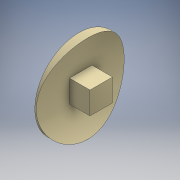
# Autodesk Inventor part: ET19
Saved by Autodesk Inventor 2016 (Build 200138000, 138)
## iProperties
Created: 2016-03-28
Part Number: ET19
Material: Genérico
Document SubType Name: Modeling
Designer: Usuario1
Density: 1 g/cm^3
Appearance: Valor por defecto
Author: Usuario1
Autodesk Inventor part; units mm, degrees
ref_plane "YZ Plane" through (0, 0, 0) normal (1, 0, 0) x (0, 1, 0)
ref_plane "XZ Plane" through (0, 0, 0) normal (0, 1, 0) x (-1, 0, 0)
ref_plane "XY Plane" through (0, 0, 0) normal (0, 0, 1) x (1, 0, 0)
sketch "Boceto1" plane through (0, 0, 0) normal (1, 0, 0) x (0, 1, 0)
  circle A0 centre (-0.0022, 0) radius 0.8492
  circle A1 centre (-1.5281, -0.0006) radius 0.1032
  circle A2 centre (0, 0) radius 0.9775
  constraints: 3 centre point
extrude "Extrusión1" add sketch "Boceto1" along normal blind 0.2 contours A0 | A2
sketch "Boceto2" plane through (0, 0, 0) normal (0, 1, 0) x (-1, 0, 0)
  arc A0 (-0.1981, -0.9764) -> (-0.1981, 0.9764) centre (-2.9972, 0) ccw
  arc A1 (-0.1981, 0.9764) -> (-0.4354, 1.174) centre (-0.4814, 0.8776) ccw
  arc A2 (-0.4354, -1.174) -> (-0.1981, -0.9764) centre (-0.4814, -0.8776) ccw
  arc A3 (-0.1981, -0.9764) -> (-0.1981, 0.9764) centre (-2.9972, 0) ccw
  arc A4 (-0.1981, 0.9764) -> (-0.4354, 1.174) centre (-0.4814, 0.8776) ccw
  arc A5 (-0.4354, -1.174) -> (-0.1981, -0.9764) centre (-0.4814, -0.8776) ccw
  arc A6 (-0.1981, -0.9764) -> (-0.1981, 0.9764) centre (-2.9972, 0) ccw
  arc A7 (-0.1981, 0.9764) -> (-0.4354, 1.174) centre (-0.4814, 0.8776) ccw
  arc A8 (-0.4354, -1.174) -> (-0.1981, -0.9764) centre (-0.4814, -0.8776) ccw
  line L0 (-0.2, 0.9775) -> (-0.2, -0.9775) projected
  line L1 (0, -0.9775) -> (0, 0.9775) projected
  line L2 (-0.4354, 1.174) -> (-0.4354, -1.174)
  point P0 (0, 0)
  constraints: 18 point on circle, 9 centre point, 2 end point, 1 vertical
extrude "Extrusión2" cut sketch "Boceto2" along normal mid plane 10
sketch "Boceto3" plane through (0, 0, 0) normal (-1, 0, 0) x (0, 0, 1)
  line L0 (0, 0) -> (0, -0.25)
  line L1 (0, -0.25) -> (-0.25, -0.25)
  line L2 (-0.25, -0.25) -> (-0.25, 0.25)
  line L3 (-0.25, 0.25) -> (0.25, 0.25)
  line L4 (0.25, 0.25) -> (0.25, -0.25)
  line L5 (0.25, -0.25) -> (-0.25, -0.25)
  dimension "d4" = 0.25
  dimension "d5" = 0.25
  dimension "d6" = 0.5
  dimension "d7" = 0.5
  dimension "d8" = 0.5
  constraints: 12 end point, 3 perpendicular, 1 point on line, 1 vertical
  measures "d4" distance of L0.start L0.end
  measures "d5" distance of L0.end L1.end
  measures "d6" distance of L1.end L2.end
  measures "d7" distance of L2.end L3.end
  measures "d8" distance of L3.end L4.end
extrude "Extrusión3" add sketch "Boceto3" against normal blind 0.5
sketch "Boceto4" plane through (0, 0, 0) normal (-1, 0, 0) x (0, 0, 1)
  line L0 (-0.9764, 0.0463) -> (-0.9764, -0.0463) projected
  line L1 (-0.9114, 0.025) -> (-0.9364, 0.025)
  line L2 (-0.9364, 0.025) -> (-0.9364, -0.025)
  line L3 (-0.9364, -0.025) -> (-0.8864, -0.025)
  line L4 (-0.8864, -0.025) -> (-0.8864, 0.025)
  line L5 (-0.8864, 0.025) -> (-0.9364, 0.025)
  line L6 (0.025, -0.9364) -> (-0.025, -0.9364)
  line L7 (-0.025, -0.9364) -> (-0.025, -0.8864)
  line L8 (-0.025, -0.8864) -> (0.025, -0.8864)
  line L9 (0.025, -0.8864) -> (0.025, -0.9364)
  line L10 (0.9114, 0.025) -> (0.9364, 0.025)
  line L11 (0.9364, 0.025) -> (0.9364, -0.025)
  line L12 (0.9364, -0.025) -> (0.8864, -0.025)
  line L13 (0.8864, -0.025) -> (0.8864, 0.025)
  line L14 (0.8864, 0.025) -> (0.9364, 0.025)
  point P0 (0, 0)
  dimension "d13" = 0.025
  dimension "d14" = 0.05
  dimension "d15" = 0.05
  dimension "d16" = 0.05
  constraints: 28 end point, 2 perpendicular, 2 point on line
  measures "d13" distance of L1.start L1.end
  measures "d14" distance of L1.end L2.end
  measures "d15" distance of L2.end L3.end
  measures "d16" distance of L3.end L4.end
extrude "Extrusión4" cut sketch "Boceto4" against normal blind 0.1 contours L5 L4 L3 L2 L1 | L10 L11 L12 L13 L14
